Autodesk Fusion 360 part; units mm, degrees
(part 2 of 2)
sketch "Sketch18" plane through (0, 10, 0) normal (0, 1, 0) x (-1, 0, 0)
  line L0 (-0.4884, 10.35) -> (2.2056, 10.35)
  line L1 (2.2056, 10.35) -> (2.2056, 6.15)
  line L2 (2.2056, 6.15) -> (-0.4884, 6.15)
  line L3 (-0.4884, 6.15) -> (-0.4884, 10.35)
  line L4 (-47.1, 4.15) -> (-47.1, 3)
  arc A0 (-47.1, 3) -> (-44.1, 0) centre (-44.1, 3) ccw
  line L5 (-44.1, 0) -> (-5.0797, 0)
  arc A1 (-5.0797, 0) -> (-2.1135, 2.5506) centre (-5.0797, 3) ccw
  line L6 (-2.1135, 2.5506) -> (-1.8712, 4.15)
  line L7 (-1.8712, 4.15) -> (1.2056, 4.15)
  line L8 (1.2056, 4.15) -> (1.2056, -1.7)
  line L9 (1.2056, -1.7) -> (0.2056, -1.7)
  line L10 (0.2056, -1.7) -> (2.7056, -6)
  line L11 (2.7056, -6) -> (2.7056, 4.15)
  line L12 (2.7056, 4.15) -> (3.2056, 4.15)
  line L13 (3.2056, 4.15) -> (3.2056, 12.35)
  line L14 (3.2056, 12.35) -> (-0.6288, 12.35)
  line L15 (-0.6288, 12.35) -> (-0.5226, 13.0506)
  arc A2 (-0.5226, 13.0506) -> (-3.4888, 16.5) centre (-3.4888, 13.5) ccw
  line L16 (-3.4888, 16.5) -> (-44.1, 16.5)
  arc A3 (-44.1, 16.5) -> (-47.1, 13.5) centre (-44.1, 13.5) ccw
  line L17 (-47.1, 13.5) -> (-47.1, 12.35)
  line L18 (-47.1, 12.35) -> (-50.7944, 12.35)
  line L19 (-50.7944, 12.35) -> (-50.7944, 4.15)
  line L20 (-50.7944, 4.15) -> (-50.2944, 4.15)
  line L21 (-50.2944, 4.15) -> (-50.2944, -6)
  line L22 (-50.2944, -6) -> (-47.7944, -1.7)
  line L23 (-47.7944, -1.7) -> (-48.7944, -1.7)
  line L24 (-48.7944, -1.7) -> (-48.7944, 4.15)
  line L25 (-48.7944, 4.15) -> (-47.1, 4.15)
  line L26 (-47.1, 6.15) -> (-49.7944, 6.15)
  line L27 (-49.7944, 6.15) -> (-49.7944, 10.35)
  line L28 (-49.7944, 10.35) -> (-47.1, 10.35)
  line L29 (-47.1, 10.35) -> (-47.1, 6.15)
  line L30 (-26.405, 10.29) -> (-26.405, 11.29)
  line L31 (-26.405, 11.29) -> (-24.005, 11.29)
  line L32 (-24.005, 11.29) -> (-24.005, 10.29)
  line L33 (-24.005, 10.29) -> (-26.405, 10.29)
  line L34 (-22.595, 10.29) -> (-22.595, 11.29)
  line L35 (-22.595, 11.29) -> (-20.195, 11.29)
  line L36 (-20.195, 11.29) -> (-20.195, 10.29)
  line L37 (-20.195, 10.29) -> (-22.595, 10.29)
  line L38 (-11.165, 10.29) -> (-11.165, 11.29)
  line L39 (-11.165, 11.29) -> (-8.765, 11.29)
  line L40 (-8.765, 11.29) -> (-8.765, 10.29)
  line L41 (-8.765, 10.29) -> (-11.165, 10.29)
  line L42 (-39.245, 11.29) -> (-39.245, 10.29)
  line L43 (-39.245, 10.29) -> (-41.645, 10.29)
  line L44 (-41.645, 10.29) -> (-41.645, 11.29)
  line L45 (-41.645, 11.29) -> (-39.245, 11.29)
  line L46 (-37.34, 6.21) -> (-37.34, 5.21)
  line L47 (-37.34, 5.21) -> (-39.74, 5.21)
  line L48 (-39.74, 5.21) -> (-39.74, 6.21)
  line L49 (-39.74, 6.21) -> (-37.34, 6.21)
  line L50 (-3.05, 6.21) -> (-3.05, 5.21)
  line L51 (-3.05, 5.21) -> (-5.45, 5.21)
  line L52 (-5.45, 5.21) -> (-5.45, 6.21)
  line L53 (-5.45, 6.21) -> (-3.05, 6.21)
  line L54 (-6.86, 6.21) -> (-6.86, 5.21)
  line L55 (-6.86, 5.21) -> (-9.26, 5.21)
  line L56 (-9.26, 5.21) -> (-9.26, 6.21)
  line L57 (-9.26, 6.21) -> (-6.86, 6.21)
  line L58 (-10.67, 6.21) -> (-10.67, 5.21)
  line L59 (-10.67, 5.21) -> (-13.07, 5.21)
  line L60 (-13.07, 5.21) -> (-13.07, 6.21)
  line L61 (-13.07, 6.21) -> (-10.67, 6.21)
  line L62 (-30.215, 10.29) -> (-30.215, 11.29)
  line L63 (-30.215, 11.29) -> (-27.815, 11.29)
  line L64 (-27.815, 11.29) -> (-27.815, 10.29)
  line L65 (-27.815, 10.29) -> (-30.215, 10.29)
  line L66 (-18.785, 10.29) -> (-18.785, 11.29)
  line L67 (-18.785, 11.29) -> (-16.385, 11.29)
  line L68 (-16.385, 11.29) -> (-16.385, 10.29)
  line L69 (-16.385, 10.29) -> (-18.785, 10.29)
  line L70 (-14.975, 10.29) -> (-14.975, 11.29)
  line L71 (-14.975, 11.29) -> (-12.575, 11.29)
  line L72 (-12.575, 11.29) -> (-12.575, 10.29)
  line L73 (-12.575, 10.29) -> (-14.975, 10.29)
  line L74 (-34.025, 10.29) -> (-34.025, 11.29)
  line L75 (-34.025, 11.29) -> (-31.625, 11.29)
  line L76 (-31.625, 11.29) -> (-31.625, 10.29)
  line L77 (-31.625, 10.29) -> (-34.025, 10.29)
  line L78 (-25.91, 6.21) -> (-25.91, 5.21)
  line L79 (-25.91, 5.21) -> (-28.31, 5.21)
  line L80 (-28.31, 5.21) -> (-28.31, 6.21)
  line L81 (-28.31, 6.21) -> (-25.91, 6.21)
  line L82 (-18.29, 6.21) -> (-18.29, 5.21)
  line L83 (-18.29, 5.21) -> (-20.69, 5.21)
  line L84 (-20.69, 5.21) -> (-20.69, 6.21)
  line L85 (-20.69, 6.21) -> (-18.29, 6.21)
  line L86 (-33.53, 6.21) -> (-33.53, 5.21)
  line L87 (-33.53, 5.21) -> (-35.93, 5.21)
  line L88 (-35.93, 5.21) -> (-35.93, 6.21)
  line L89 (-35.93, 6.21) -> (-33.53, 6.21)
  line L90 (-41.15, 6.21) -> (-41.15, 5.21)
  line L91 (-41.15, 5.21) -> (-43.55, 5.21)
  line L92 (-43.55, 5.21) -> (-43.55, 6.21)
  line L93 (-43.55, 6.21) -> (-41.15, 6.21)
  line L94 (-14.48, 6.21) -> (-14.48, 5.21)
  line L95 (-14.48, 5.21) -> (-16.88, 5.21)
  line L96 (-16.88, 5.21) -> (-16.88, 6.21)
  line L97 (-16.88, 6.21) -> (-14.48, 6.21)
  line L98 (-37.835, 10.29) -> (-37.835, 11.29)
  line L99 (-37.835, 11.29) -> (-35.435, 11.29)
  line L100 (-35.435, 11.29) -> (-35.435, 10.29)
  line L101 (-35.435, 10.29) -> (-37.835, 10.29)
  line L102 (-7.355, 10.29) -> (-7.355, 11.29)
  line L103 (-7.355, 11.29) -> (-4.955, 11.29)
  line L104 (-4.955, 11.29) -> (-4.955, 10.29)
  line L105 (-4.955, 10.29) -> (-7.355, 10.29)
  line L106 (-29.72, 6.21) -> (-29.72, 5.21)
  line L107 (-29.72, 5.21) -> (-32.12, 5.21)
  line L108 (-32.12, 5.21) -> (-32.12, 6.21)
  line L109 (-32.12, 6.21) -> (-29.72, 6.21)
  line L110 (-22.1, 6.21) -> (-22.1, 5.21)
  line L111 (-22.1, 5.21) -> (-24.5, 5.21)
  line L112 (-24.5, 5.21) -> (-24.5, 6.21)
  line L113 (-24.5, 6.21) -> (-22.1, 6.21)
  line L114 (-42.35, 5.21) -> (-42.35, 0) construction
  line L115 (-43.05, 5.21) -> (-43.05, 0)
  line L116 (-41.65, 5.21) -> (-41.65, 0)
  line L117 (-37.84, 5.21) -> (-37.84, 0)
  line L118 (-39.24, 5.21) -> (-39.24, 0)
  line L119 (-34.03, 5.21) -> (-34.03, 0)
  line L120 (-35.43, 5.21) -> (-35.43, 0)
  line L121 (-30.22, 5.21) -> (-30.22, 0)
  line L122 (-31.62, 5.21) -> (-31.62, 0)
  line L123 (-26.41, 5.21) -> (-26.41, 0)
  line L124 (-27.81, 5.21) -> (-27.81, 0)
  line L125 (-22.6, 5.21) -> (-22.6, 0)
  line L126 (-24, 5.21) -> (-24, 0)
  line L127 (-18.79, 5.21) -> (-18.79, 0)
  line L128 (-20.19, 5.21) -> (-20.19, 0)
  line L129 (-14.98, 5.21) -> (-14.98, 0)
  line L130 (-16.38, 5.21) -> (-16.38, 0)
  line L131 (-11.17, 5.21) -> (-11.17, 0)
  line L132 (-12.57, 5.21) -> (-12.57, 0)
  line L133 (-7.36, 5.21) -> (-7.36, 0)
  line L134 (-8.76, 5.21) -> (-8.76, 0)
  line L135 (-3.55, 5.21) -> (-3.55, 0)
  line L136 (-4.95, 5.21) -> (-4.95, 0)
  line L137 (-3.55, 0) -> (-5.0797, 0)
  dimension "d118" = 0.7
  dimension "d119" = -0.7
  dimension "d122" = 3.81
  dimension "d123" = 0
  constraint midpoint L91 L114.start
  constraint coincident L5 L114.end
  constraint perpendicular L5 L114
  constraint coincident L5.end A1.start
  constraint tangent A1 L137
extrude "Extrude14" add sketch "Sketch18" along normal blind 5.1 contours L5 L91 L115 L116 | L5 L47 L117 L118 | L5 L87 L119 L120 | L5 L107 L121 L122 | L5 L79 L123 L124 | L5 L111 L125 L126 | L5 L83 L127 L128 | L5 L95 L129 L130 | L5 L59 L131 L132 | L5 L55 L133 L134 | A1 L135 L136 L137 | A1 L51 L135 L136 bodies 1
sketch "Sketch20" plane through (43.05, 0, 0) normal (1, 0, 0) x (0, 1, 0)
  line L0 (10, 5.21) -> (10, 0)
  line L1 (10, 0) -> (15.1, 0)
  line L2 (15.1, 0) -> (15.1, 5.21)
  line L3 (15.1, 5.21) -> (10, 5.21)
  line L4 (10, 5.21) -> (14.4, 5.21)
  line L5 (15.1, 4.51) -> (15.1, 2.3)
  arc A0 (15.1, 4.51) -> (14.4, 5.21) centre (14.4, 4.51) ccw
  dimension "d132" = 0.7
  constraint coincident L0.start L3.end
  constraint coincident L2 L5.end
  constraint perpendicular L3 L5
  constraint tangent L4 A0
  constraint tangent L5 A0
  measures "d132" radius of A0
fillet "Fillet9" radius 0.2 11 edges at (42.35, 15.1, 5.21) (38.54, 15.1, 5.21) (34.73, 15.1, 5.21) (30.92, 15.1, 5.21) (27.11, 15.1, 5.21) (23.3, 15.1, 5.21) (19.49, 15.1, 5.21) (15.68, 15.1, 5.21) (11.87, 15.1, 5.21) (8.06, 15.1, 5.21) (4.25, 15.1, 5.21) on bodies 1
sketch "Sketch15" plane through (0, 10, 0) normal (0, 1, 0) x (-1, 0, 0)
  line L0 (-0.4884, 10.35) -> (2.2056, 10.35)
  line L1 (2.2056, 10.35) -> (2.2056, 6.15)
  line L2 (2.2056, 6.15) -> (-0.4884, 6.15)
  line L3 (-0.4884, 6.15) -> (-0.4884, 10.35)
  line L4 (-47.1, 4.15) -> (-47.1, 3)
  arc A0 (-47.1, 3) -> (-44.1, 0) centre (-44.1, 3) ccw
  line L5 (-41.65, 0) -> (-39.24, 0)
  arc A1 (-5.0797, 0) -> (-4.95, 0.0028) centre (-5.0797, 3) ccw
  line L6 (-2.1135, 2.5506) -> (-1.8712, 4.15)
  line L7 (-1.8712, 4.15) -> (1.2056, 4.15)
  line L8 (1.2056, 4.15) -> (1.2056, -1.7)
  line L9 (1.2056, -1.7) -> (0.2056, -1.7)
  line L10 (0.2056, -1.7) -> (2.7056, -6)
  line L11 (2.7056, -6) -> (2.7056, 4.15)
  line L12 (2.7056, 4.15) -> (3.2056, 4.15)
  line L13 (3.2056, 4.15) -> (3.2056, 12.35)
  line L14 (3.2056, 12.35) -> (-0.6288, 12.35)
  line L15 (-0.6288, 12.35) -> (-0.5226, 13.0506)
  arc A2 (-0.5226, 13.0506) -> (-3.4888, 16.5) centre (-3.4888, 13.5) ccw
  line L16 (-3.4888, 16.5) -> (-44.1, 16.5)
  arc A3 (-44.1, 16.5) -> (-47.1, 13.5) centre (-44.1, 13.5) ccw
  line L17 (-47.1, 13.5) -> (-47.1, 12.35)
  line L18 (-47.1, 12.35) -> (-50.7944, 12.35)
  line L19 (-50.7944, 12.35) -> (-50.7944, 4.15)
  line L20 (-50.7944, 4.15) -> (-50.2944, 4.15)
  line L21 (-50.2944, 4.15) -> (-50.2944, -6)
  line L22 (-50.2944, -6) -> (-47.7944, -1.7)
  line L23 (-47.7944, -1.7) -> (-48.7944, -1.7)
  line L24 (-48.7944, -1.7) -> (-48.7944, 4.15)
  line L25 (-48.7944, 4.15) -> (-47.1, 4.15)
  line L26 (-47.1, 6.15) -> (-49.7944, 6.15)
  line L27 (-49.7944, 6.15) -> (-49.7944, 10.35)
  line L28 (-49.7944, 10.35) -> (-47.1, 10.35)
  line L29 (-47.1, 10.35) -> (-47.1, 6.15)
  line L30 (-26.405, 10.29) -> (-26.405, 11.29)
  line L31 (-26.405, 11.29) -> (-24.005, 11.29)
  line L32 (-24.005, 11.29) -> (-24.005, 10.29)
  line L33 (-24.005, 10.29) -> (-26.405, 10.29)
  line L34 (-22.595, 10.29) -> (-22.595, 11.29)
  line L35 (-22.595, 11.29) -> (-20.195, 11.29)
  line L36 (-20.195, 11.29) -> (-20.195, 10.29)
  line L37 (-20.195, 10.29) -> (-22.595, 10.29)
  line L38 (-11.165, 10.29) -> (-11.165, 11.29)
  line L39 (-11.165, 11.29) -> (-8.765, 11.29)
  line L40 (-8.765, 11.29) -> (-8.765, 10.29)
  line L41 (-8.765, 10.29) -> (-11.165, 10.29)
  line L42 (-39.245, 11.29) -> (-39.245, 10.29)
  line L43 (-39.245, 10.29) -> (-41.645, 10.29)
  line L44 (-41.645, 10.29) -> (-41.645, 11.29)
  line L45 (-41.645, 11.29) -> (-39.245, 11.29)
  line L46 (-37.34, 6.21) -> (-37.34, 5.21)
  line L47 (-39.24, 5.21) -> (-39.74, 5.21)
  line L48 (-39.74, 5.21) -> (-39.74, 6.21)
  line L49 (-39.74, 6.21) -> (-37.34, 6.21)
  line L50 (-3.05, 6.21) -> (-3.05, 5.21)
  line L51 (-4.95, 5.21) -> (-5.45, 5.21)
  line L52 (-5.45, 5.21) -> (-5.45, 6.21)
  line L53 (-5.45, 6.21) -> (-3.05, 6.21)
  line L54 (-6.86, 6.21) -> (-6.86, 5.21)
  line L55 (-8.76, 5.21) -> (-9.26, 5.21)
  line L56 (-9.26, 5.21) -> (-9.26, 6.21)
  line L57 (-9.26, 6.21) -> (-6.86, 6.21)
  line L58 (-10.67, 6.21) -> (-10.67, 5.21)
  line L59 (-12.57, 5.21) -> (-13.07, 5.21)
  line L60 (-13.07, 5.21) -> (-13.07, 6.21)
  line L61 (-13.07, 6.21) -> (-10.67, 6.21)
  line L62 (-30.215, 10.29) -> (-30.215, 11.29)
  line L63 (-30.215, 11.29) -> (-27.815, 11.29)
  line L64 (-27.815, 11.29) -> (-27.815, 10.29)
  line L65 (-27.815, 10.29) -> (-30.215, 10.29)
  line L66 (-18.785, 10.29) -> (-18.785, 11.29)
  line L67 (-18.785, 11.29) -> (-16.385, 11.29)
  line L68 (-16.385, 11.29) -> (-16.385, 10.29)
  line L69 (-16.385, 10.29) -> (-18.785, 10.29)
  line L70 (-14.975, 10.29) -> (-14.975, 11.29)
  line L71 (-14.975, 11.29) -> (-12.575, 11.29)
  line L72 (-12.575, 11.29) -> (-12.575, 10.29)
  line L73 (-12.575, 10.29) -> (-14.975, 10.29)
  line L74 (-34.025, 10.29) -> (-34.025, 11.29)
  line L75 (-34.025, 11.29) -> (-31.625, 11.29)
  line L76 (-31.625, 11.29) -> (-31.625, 10.29)
  line L77 (-31.625, 10.29) -> (-34.025, 10.29)
  line L78 (-25.91, 6.21) -> (-25.91, 5.21)
  line L79 (-27.81, 5.21) -> (-28.31, 5.21)
  line L80 (-28.31, 5.21) -> (-28.31, 6.21)
  line L81 (-28.31, 6.21) -> (-25.91, 6.21)
  line L82 (-18.29, 6.21) -> (-18.29, 5.21)
  line L83 (-20.19, 5.21) -> (-20.69, 5.21)
  line L84 (-20.69, 5.21) -> (-20.69, 6.21)
  line L85 (-20.69, 6.21) -> (-18.29, 6.21)
  line L86 (-33.53, 6.21) -> (-33.53, 5.21)
  line L87 (-35.43, 5.21) -> (-35.93, 5.21)
  line L88 (-35.93, 5.21) -> (-35.93, 6.21)
  line L89 (-35.93, 6.21) -> (-33.53, 6.21)
  line L90 (-41.15, 6.21) -> (-41.15, 5.21)
  line L91 (-43.05, 5.21) -> (-43.55, 5.21)
  line L92 (-43.55, 5.21) -> (-43.55, 6.21)
  line L93 (-43.55, 6.21) -> (-41.15, 6.21)
  line L94 (-14.48, 6.21) -> (-14.48, 5.21)
  line L95 (-16.38, 5.21) -> (-16.88, 5.21)
  line L96 (-16.88, 5.21) -> (-16.88, 6.21)
  line L97 (-16.88, 6.21) -> (-14.48, 6.21)
  line L98 (-37.835, 10.29) -> (-37.835, 11.29)
  line L99 (-37.835, 11.29) -> (-35.435, 11.29)
  line L100 (-35.435, 11.29) -> (-35.435, 10.29)
  line L101 (-35.435, 10.29) -> (-37.835, 10.29)
  line L102 (-7.355, 10.29) -> (-7.355, 11.29)
  line L103 (-7.355, 11.29) -> (-4.955, 11.29)
  line L104 (-4.955, 11.29) -> (-4.955, 10.29)
  line L105 (-4.955, 10.29) -> (-7.355, 10.29)
  line L106 (-29.72, 6.21) -> (-29.72, 5.21)
  line L107 (-31.62, 5.21) -> (-32.12, 5.21)
  line L108 (-32.12, 5.21) -> (-32.12, 6.21)
  line L109 (-32.12, 6.21) -> (-29.72, 6.21)
  line L110 (-22.1, 6.21) -> (-22.1, 5.21)
  line L111 (-24, 5.21) -> (-24.5, 5.21)
  line L112 (-24.5, 5.21) -> (-24.5, 6.21)
  line L113 (-24.5, 6.21) -> (-22.1, 6.21)
  line L114 (-41.545, 10.99) -> (-39.345, 10.99)
  line L115 (-39.345, 10.99) -> (-39.345, 10.59)
  line L116 (-39.345, 10.59) -> (-41.545, 10.59)
  line L117 (-41.545, 10.59) -> (-41.545, 10.99)
  line L118 (-41.65, 5.21) -> (-41.65, 0)
  line L119 (-39.24, 0) -> (-39.24, 5.21)
  line L120 (-37.34, 5.21) -> (-37.84, 5.21)
  line L121 (-37.84, 5.21) -> (-37.84, 0)
  line L122 (-37.84, 0) -> (-35.43, 0)
  line L123 (-35.43, 0) -> (-35.43, 5.21)
  line L124 (-33.53, 5.21) -> (-34.03, 5.21)
  line L125 (-34.03, 5.21) -> (-34.03, 0)
  line L126 (-34.03, 0) -> (-31.62, 0)
  line L127 (-31.62, 0) -> (-31.62, 5.21)
  line L128 (-29.72, 5.21) -> (-30.22, 5.21)
  line L129 (-30.22, 5.21) -> (-30.22, 0)
  line L130 (-30.22, 0) -> (-27.81, 0)
  line L131 (-27.81, 0) -> (-27.81, 5.21)
  line L132 (-25.91, 5.21) -> (-26.41, 5.21)
  line L133 (-26.41, 5.21) -> (-26.41, 0)
  line L134 (-26.41, 0) -> (-24, 0)
  line L135 (-24, 0) -> (-24, 5.21)
  line L136 (-22.1, 5.21) -> (-22.6, 5.21)
  line L137 (-22.6, 5.21) -> (-22.6, 0)
  line L138 (-22.6, 0) -> (-20.19, 0)
  line L139 (-20.19, 0) -> (-20.19, 5.21)
  line L140 (-18.29, 5.21) -> (-18.79, 5.21)
  line L141 (-18.79, 5.21) -> (-18.79, 0)
  line L142 (-18.79, 0) -> (-16.38, 0)
  line L143 (-16.38, 0) -> (-16.38, 5.21)
  line L144 (-14.48, 5.21) -> (-14.98, 5.21)
  line L145 (-14.98, 5.21) -> (-14.98, 0)
  line L146 (-14.98, 0) -> (-12.57, 0)
  line L147 (-12.57, 0) -> (-12.57, 5.21)
  line L148 (-10.67, 5.21) -> (-11.17, 5.21)
  line L149 (-11.17, 5.21) -> (-11.17, 0)
  line L150 (-11.17, 0) -> (-8.76, 0)
  line L151 (-8.76, 0) -> (-8.76, 5.21)
  line L152 (-6.86, 5.21) -> (-7.36, 5.21)
  line L153 (-7.36, 5.21) -> (-7.36, 0)
  line L154 (-7.36, 0) -> (-5.0797, 0)
  line L155 (-4.95, 0.0028) -> (-4.95, 5.21)
  line L156 (-3.05, 5.21) -> (-3.55, 5.21)
  line L157 (-3.55, 5.21) -> (-3.55, 0.4193)
  arc A4 (-3.55, 0.4193) -> (-2.1135, 2.5506) centre (-5.0797, 3) ccw
  line L158 (-44.1, 0) -> (-43.05, 0)
  line L159 (-43.05, 0) -> (-43.05, 5.21)
  line L160 (-41.15, 5.21) -> (-41.65, 5.21)
  dimension "d88" = 0.1
  dimension "d89" = 0.1
  dimension "d90" = 0.3
  dimension "d91" = 0.3
  constraint horizontal L114
  constraint vertical L115
  constraint horizontal L116
  constraint vertical L117
  measures "d88" distance of L42 L115
  measures "d89" distance of L44 L117
  measures "d90" distance of L45 L114
  measures "d91" distance of L43 L116
extrude "Extrude11" add sketch "Sketch15" against normal blind 10 separate body contours L114 L115 L116 L117 makes body 2
sketch "Sketch16" plane through (0, 0, 10.99) normal (0, 0, 1) x (-1, 0, 0)
  line L0 (-41.545, -10) -> (-39.345, -10)
  line L1 (-39.345, -10) -> (-39.345, 0)
  line L2 (-39.345, 0) -> (-41.545, 0)
  line L3 (-41.545, 0) -> (-41.545, -10)
  line L4 (-39.745, 0) -> (-41.145, 0)
  line L5 (-41.145, 0) -> (-41.145, -7)
  line L6 (-41.145, -7) -> (-39.745, -7)
  line L7 (-39.745, -7) -> (-39.745, 0)
  dimension "d94" = 7
  dimension "d95" = 0.4
  dimension "d96" = 0.4
  constraint horizontal L4
  constraint vertical L5
  constraint horizontal L6
  constraint vertical L7
  constraint coincident L2 L4.start
  measures "d94" distance of L4.start L6.end
  measures "d95" distance of L1 L7
  measures "d96" distance of L3 L5
extrude "Extrude12" cut sketch "Sketch16" against normal through all contours L2 L4 L5 L6 L7 bodies 2
sketch "Sketch17" plane through (0, 10, 0) normal (0, 1, 0) x (-1, 0, 0)
  line L0 (-41.545, 10.59) -> (-39.345, 10.59)
  line L1 (-39.345, 10.59) -> (-39.345, 10.99)
  line L2 (-39.345, 10.99) -> (-41.545, 10.99)
  line L3 (-41.545, 10.99) -> (-41.545, 10.59)
  line L4 (-41.545, 10.99) -> (-39.345, 10.99)
  line L5 (-39.345, 10.99) -> (-39.345, -4.5)
  line L6 (-39.345, -4.5) -> (-41.545, -4.5)
  line L7 (-41.545, -4.5) -> (-41.545, 10.99)
  line L8 (-40.445, -4.5) -> (-40.445, 10.99) construction
  line L9 (-40.045, -4.5) -> (-40.045, 10.99)
  line L10 (-40.845, -4.5) -> (-40.845, 10.99)
  line L11 (-40.845, 6.71) -> (-41.545, 7.41)
  line L12 (-40.845, 6.71) -> (-39.8551, 6.71) construction
  line L13 (-40.045, 6.71) -> (-39.345, 7.41)
  line L14 (-40.845, 4.71) -> (-41.545, 4.01)
  line L15 (-40.845, 4.71) -> (-39.8551, 4.71) construction
  line L16 (-40.045, 4.71) -> (-39.345, 4.01)
  line L17 (-40.845, 0) -> (-41.545, 0.7)
  line L18 (-40.045, 0) -> (-39.345, 0.7)
  line L19 (-39.645, 10.99) -> (-39.645, -4.5)
  line L20 (-41.245, -4.5) -> (-41.245, 10.99)
  line L21 (-40.445, -4.5) -> (-40.045, -4.1)
  line L22 (-40.445, -4.5) -> (-39.8793, -4.5) construction
  line L23 (-40.445, -4.5) -> (-40.845, -4.1)
  line L24 (-7.36, 0) -> (-5.0797, 0)
  line L25 (-11.17, 0) -> (-8.76, 0)
  line L26 (-14.98, 0) -> (-12.57, 0)
  line L27 (-18.79, 0) -> (-16.38, 0)
  line L28 (-22.6, 0) -> (-20.19, 0)
  line L29 (-26.41, 0) -> (-24, 0)
  line L30 (-30.22, 0) -> (-27.81, 0)
  line L31 (-34.03, 0) -> (-31.62, 0)
  line L32 (-37.84, 0) -> (-35.43, 0)
  line L33 (-41.65, 0) -> (-39.24, 0)
  line L34 (-43.05, 5.21) -> (-43.55, 5.21)
  line L35 (-44.1, 0) -> (-43.05, 0)
  line L36 (-41.15, 5.21) -> (-41.65, 5.21)
  line L37 (-40.845, 10.99) -> (-40.2793, 10.99) construction
  line L38 (-40.845, 10.59) -> (-41.245, 10.19)
  line L39 (-40.845, 10.59) -> (-40.2793, 10.59) construction
  line L40 (-40.045, 10.59) -> (-39.645, 10.19)
  point P0 (-41.15, 6.21)
  dimension "d99" = 0.4
  dimension "d100" = -0.4
  dimension "d101" = 135
  dimension "d102" = 0.5
  dimension "d103" = 135
  dimension "d104" = 0.9899
  dimension "d106" = 0.3
  dimension "d107" = 0.3
  dimension "d110" = 45
  dimension "d158" = 135
  constraint horizontal L4
  constraint vertical L5
  constraint horizontal L6
  constraint vertical L7
  constraint coincident L2.end L3.start
  constraint midpoint L6 L8.start
  constraint midpoint L4 L8.end
  constraint horizontal L12
  constraint coincident L10 L11.start
  constraint coincident L7 L11.end
  constraint coincident L12 L13.start
  constraint coincident L9 L13.start
  constraint coincident L5 L13.end
  constraint perpendicular L11 L13
  constraint horizontal L15
  constraint coincident L10 L14.start
  constraint coincident L7 L14.end
  constraint coincident L9 L16.start
  constraint coincident L15 L16.start
  constraint coincident L5 L16.end
  constraint coincident L10 L17.start
  constraint coincident L7 L17.end
  constraint parallel L16 L17
  constraint coincident L9 L18.start
  constraint coincident L5 L18.end
  constraint perpendicular L17 L18
  constraint horizontal L22
  constraint coincident L9 L21.end
  constraint coincident L10 L23.end
  constraint perpendicular L21 L23
  constraint horizontal L37
  constraint horizontal L39
  constraint coincident L0 L38.start
  constraint coincident L10 L38.start
  constraint coincident L20 L38.end
  constraint coincident L9 L40.start
  constraint coincident L0 L40.start
  constraint coincident L19 L40.end
  constraint perpendicular L38 L40
  measures "d101" angle of L11 L12
  measures "d102" vertical distance of L11.start P0
  measures "d103" angle of L14 L15
  measures "d104" distance of L14.start L15.end
  measures "d110" angle of L21 L22
  measures "d158" angle of L38 L39
extrude "Extrude13" add sketch "Sketch17" along normal blind 0.4 contours L0 L2 L4 L9 L10 | L0 L9 L10 L33 | L10 L11 L20 L38 | L9 L13 L19 L40 | L10 L14 L17 L20 | L9 L16 L18 L19 | L9 L10 L21 L23 L33 bodies 2
fillet "Fillet8" radius 0.2 23 edges at (39.745, 0, 10.79) (41.145, 0, 10.79) (39.345, 10, 10.79) (41.545, 10, 10.79) (40.445, 10.4, 10.99) (39.645, 10.2, 7.11) (40.045, 10.2, 6.71) (40.045, 10.2, 4.71) (39.645, 10.2, 4.31) (41.245, 10.2, 7.11) (40.845, 10.2, 6.71) (40.845, 10.2, 4.71) (41.245, 10.2, 4.31) (41.245, 10.2, 0.4) (39.645, 10.2, 0.4) (40.045, 10.2, -4.1) (40.845, 10.2, -4.1) (41.245, 10.2, 10.19) (40.845, 10.2, 10.59) (39.645, 10.2, 10.19) (40.045, 10.2, 10.59) (40.845, 10.2, 0) (40.045, 10.2, 0) on bodies 2
pattern_linear "R-Pattern1" count 10 spacing 3.81 along (-1, 0, 0) of bodies 2 makes body 3 at (36.3683, 10.4, 2.9791) makes body 4 at (32.5583, 10.4, 2.9791) makes body 5 at (28.7483, 10.4, 2.9791) makes body 6 at (24.9383, 10.4, 2.9791) makes body 7 at (21.1283, 10.4, 2.9791) makes body 8 at (17.3183, 10.4, 2.9791) makes body 9 at (13.5083, 10.4, 2.9791) makes body 10 at (9.6983, 10.4, 2.9791) makes body 11 at (5.8883, 10.4, 2.9791)
sketch "Sketch19" plane through (0, 10, 0) normal (0, 1, 0) x (-1, 0, 0)
  line L0 (-41.65, 5.21) -> (-41.65, 0)
  line L1 (-41.65, 0) -> (-39.24, 0)
  line L2 (-39.24, 0) -> (-39.24, 5.21)
  line L3 (-39.24, 5.21) -> (-39.74, 5.21)
  line L4 (-39.74, 5.21) -> (-39.74, 6.21)
  line L5 (-39.74, 6.21) -> (-37.34, 6.21)
  line L6 (-37.34, 6.21) -> (-37.34, 5.21)
  line L7 (-37.34, 5.21) -> (-37.84, 5.21)
  line L8 (-37.84, 5.21) -> (-37.84, 0)
  line L9 (-37.84, 0) -> (-35.43, 0)
  line L10 (-35.43, 0) -> (-35.43, 5.21)
  line L11 (-35.43, 5.21) -> (-35.93, 5.21)
  line L12 (-35.93, 5.21) -> (-35.93, 6.21)
  line L13 (-35.93, 6.21) -> (-33.53, 6.21)
  line L14 (-33.53, 6.21) -> (-33.53, 5.21)
  line L15 (-33.53, 5.21) -> (-34.03, 5.21)
  line L16 (-34.03, 5.21) -> (-34.03, 0)
  line L17 (-34.03, 0) -> (-31.62, 0)
  line L18 (-31.62, 0) -> (-31.62, 5.21)
  line L19 (-31.62, 5.21) -> (-32.12, 5.21)
  line L20 (-32.12, 5.21) -> (-32.12, 6.21)
  line L21 (-32.12, 6.21) -> (-29.72, 6.21)
  line L22 (-29.72, 6.21) -> (-29.72, 5.21)
  line L23 (-29.72, 5.21) -> (-30.22, 5.21)
  line L24 (-30.22, 5.21) -> (-30.22, 0)
  line L25 (-30.22, 0) -> (-27.81, 0)
  line L26 (-27.81, 0) -> (-27.81, 5.21)
  line L27 (-27.81, 5.21) -> (-28.31, 5.21)
  line L28 (-28.31, 5.21) -> (-28.31, 6.21)
  line L29 (-28.31, 6.21) -> (-25.91, 6.21)
  line L30 (-25.91, 6.21) -> (-25.91, 5.21)
  line L31 (-25.91, 5.21) -> (-26.41, 5.21)
  line L32 (-26.41, 5.21) -> (-26.41, 0)
  line L33 (-26.41, 0) -> (-24, 0)
  line L34 (-24, 0) -> (-24, 5.21)
  line L35 (-24, 5.21) -> (-24.5, 5.21)
  line L36 (-24.5, 5.21) -> (-24.5, 6.21)
  line L37 (-24.5, 6.21) -> (-22.1, 6.21)
  line L38 (-22.1, 6.21) -> (-22.1, 5.21)
  line L39 (-22.1, 5.21) -> (-22.6, 5.21)
  line L40 (-22.6, 5.21) -> (-22.6, 0)
  line L41 (-22.6, 0) -> (-20.19, 0)
  line L42 (-20.19, 0) -> (-20.19, 5.21)
  line L43 (-20.19, 5.21) -> (-20.69, 5.21)
  line L44 (-20.69, 5.21) -> (-20.69, 6.21)
  line L45 (-20.69, 6.21) -> (-18.29, 6.21)
  line L46 (-18.29, 6.21) -> (-18.29, 5.21)
  line L47 (-18.29, 5.21) -> (-18.79, 5.21)
  line L48 (-18.79, 5.21) -> (-18.79, 0)
  line L49 (-18.79, 0) -> (-16.38, 0)
  line L50 (-16.38, 0) -> (-16.38, 5.21)
  line L51 (-16.38, 5.21) -> (-16.88, 5.21)
  line L52 (-16.88, 5.21) -> (-16.88, 6.21)
  line L53 (-16.88, 6.21) -> (-14.48, 6.21)
  line L54 (-14.48, 6.21) -> (-14.48, 5.21)
  line L55 (-14.48, 5.21) -> (-14.98, 5.21)
  line L56 (-14.98, 5.21) -> (-14.98, 0)
  line L57 (-14.98, 0) -> (-12.57, 0)
  line L58 (-12.57, 0) -> (-12.57, 5.21)
  line L59 (-12.57, 5.21) -> (-13.07, 5.21)
  line L60 (-13.07, 5.21) -> (-13.07, 6.21)
  line L61 (-13.07, 6.21) -> (-10.67, 6.21)
  line L62 (-10.67, 6.21) -> (-10.67, 5.21)
  line L63 (-10.67, 5.21) -> (-11.17, 5.21)
  line L64 (-11.17, 5.21) -> (-11.17, 0)
  line L65 (-11.17, 0) -> (-8.76, 0)
  line L66 (-8.76, 0) -> (-8.76, 5.21)
  line L67 (-8.76, 5.21) -> (-9.26, 5.21)
  line L68 (-9.26, 5.21) -> (-9.26, 6.21)
  line L69 (-9.26, 6.21) -> (-6.86, 6.21)
  line L70 (-6.86, 6.21) -> (-6.86, 5.21)
  line L71 (-6.86, 5.21) -> (-7.36, 5.21)
  line L72 (-7.36, 5.21) -> (-7.36, 0)
  line L73 (-7.36, 0) -> (-5.0797, 0)
  arc A0 (-5.0797, 0) -> (-4.95, 0.0028) centre (-5.0797, 3) ccw
  line L74 (-4.95, 0.0028) -> (-4.95, 5.21)
  line L75 (-4.95, 5.21) -> (-5.45, 5.21)
  line L76 (-5.45, 5.21) -> (-5.45, 6.21)
  line L77 (-5.45, 6.21) -> (-3.05, 6.21)
  line L78 (-3.05, 6.21) -> (-3.05, 5.21)
  line L79 (-3.05, 5.21) -> (-3.55, 5.21)
  line L80 (-3.55, 5.21) -> (-3.55, 0.4193)
  arc A1 (-3.55, 0.4193) -> (-2.1135, 2.5506) centre (-5.0797, 3) ccw
  line L81 (-2.1135, 2.5506) -> (-1.8712, 4.15)
  line L82 (-1.8712, 4.15) -> (1.2056, 4.15)
  line L83 (1.2056, 4.15) -> (1.2056, -1.7)
  line L84 (1.2056, -1.7) -> (0.2056, -1.7)
  line L85 (0.2056, -1.7) -> (2.7056, -6)
  line L86 (2.7056, -6) -> (2.7056, 4.15)
  line L87 (2.7056, 4.15) -> (3.2056, 4.15)
  line L88 (3.2056, 4.15) -> (3.2056, 12.35)
  line L89 (3.2056, 12.35) -> (-0.6288, 12.35)
  line L90 (-0.6288, 12.35) -> (-0.5226, 13.0506)
  arc A2 (-0.5226, 13.0506) -> (-3.4888, 16.5) centre (-3.4888, 13.5) ccw
  line L91 (-3.4888, 16.5) -> (-44.1, 16.5)
  arc A3 (-44.1, 16.5) -> (-47.1, 13.5) centre (-44.1, 13.5) ccw
  line L92 (-47.1, 13.5) -> (-47.1, 12.35)
  line L93 (-47.1, 12.35) -> (-50.7944, 12.35)
  line L94 (-50.7944, 12.35) -> (-50.7944, 4.15)
  line L95 (-50.7944, 4.15) -> (-50.2944, 4.15)
  line L96 (-50.2944, 4.15) -> (-50.2944, -6)
  line L97 (-50.2944, -6) -> (-47.7944, -1.7)
  line L98 (-47.7944, -1.7) -> (-48.7944, -1.7)
  line L99 (-48.7944, -1.7) -> (-48.7944, 4.15)
  line L100 (-48.7944, 4.15) -> (-47.1, 4.15)
  line L101 (-47.1, 4.15) -> (-47.1, 3)
  arc A4 (-47.1, 3) -> (-44.1, 0) centre (-44.1, 3) ccw
  line L102 (-44.1, 0) -> (-43.05, 0)
  line L103 (-43.05, 0) -> (-43.05, 5.21)
  line L104 (-43.05, 5.21) -> (-43.55, 5.21)
  line L105 (-43.55, 5.21) -> (-43.55, 6.21)
  line L106 (-43.55, 6.21) -> (-41.15, 6.21)
  line L107 (-41.15, 6.21) -> (-41.15, 5.21)
  line L108 (-41.15, 5.21) -> (-41.65, 5.21)
  line L109 (-0.4884, 10.35) -> (2.2056, 10.35)
  line L110 (2.2056, 10.35) -> (2.2056, 6.15)
  line L111 (2.2056, 6.15) -> (-0.4884, 6.15)
  line L112 (-0.4884, 6.15) -> (-0.4884, 10.35)
  line L113 (-47.1, 6.15) -> (-49.7944, 6.15)
  line L114 (-49.7944, 6.15) -> (-49.7944, 10.35)
  line L115 (-49.7944, 10.35) -> (-47.1, 10.35)
  line L116 (-47.1, 10.35) -> (-47.1, 6.15)
  line L117 (-26.405, 10.29) -> (-26.405, 11.29)
  line L118 (-26.405, 11.29) -> (-24.005, 11.29)
  line L119 (-24.005, 11.29) -> (-24.005, 10.29)
  line L120 (-24.005, 10.29) -> (-26.405, 10.29)
  line L121 (-22.595, 10.29) -> (-22.595, 11.29)
  line L122 (-22.595, 11.29) -> (-20.195, 11.29)
  line L123 (-20.195, 11.29) -> (-20.195, 10.29)
  line L124 (-20.195, 10.29) -> (-22.595, 10.29)
  line L125 (-11.165, 10.29) -> (-11.165, 11.29)
  line L126 (-11.165, 11.29) -> (-8.765, 11.29)
  line L127 (-8.765, 11.29) -> (-8.765, 10.29)
  line L128 (-8.765, 10.29) -> (-11.165, 10.29)
  line L129 (-39.245, 11.29) -> (-39.245, 10.29)
  line L130 (-39.245, 10.29) -> (-41.645, 10.29)
  line L131 (-41.645, 10.29) -> (-41.645, 11.29)
  line L132 (-41.645, 11.29) -> (-39.245, 11.29)
  line L133 (-30.215, 10.29) -> (-30.215, 11.29)
  line L134 (-30.215, 11.29) -> (-27.815, 11.29)
  line L135 (-27.815, 11.29) -> (-27.815, 10.29)
  line L136 (-27.815, 10.29) -> (-30.215, 10.29)
  line L137 (-18.785, 10.29) -> (-18.785, 11.29)
  line L138 (-18.785, 11.29) -> (-16.385, 11.29)
  line L139 (-16.385, 11.29) -> (-16.385, 10.29)
  line L140 (-16.385, 10.29) -> (-18.785, 10.29)
  line L141 (-14.975, 10.29) -> (-14.975, 11.29)
  line L142 (-14.975, 11.29) -> (-12.575, 11.29)
  line L143 (-12.575, 11.29) -> (-12.575, 10.29)
  line L144 (-12.575, 10.29) -> (-14.975, 10.29)
  line L145 (-34.025, 10.29) -> (-34.025, 11.29)
  line L146 (-34.025, 11.29) -> (-31.625, 11.29)
  line L147 (-31.625, 11.29) -> (-31.625, 10.29)
  line L148 (-31.625, 10.29) -> (-34.025, 10.29)
  line L149 (-37.835, 10.29) -> (-37.835, 11.29)
  line L150 (-37.835, 11.29) -> (-35.435, 11.29)
  line L151 (-35.435, 11.29) -> (-35.435, 10.29)
  line L152 (-35.435, 10.29) -> (-37.835, 10.29)
  line L153 (-7.355, 10.29) -> (-7.355, 11.29)
  line L154 (-7.355, 11.29) -> (-4.955, 11.29)
  line L155 (-4.955, 11.29) -> (-4.955, 10.29)
  line L156 (-4.955, 10.29) -> (-7.355, 10.29)
  line L157 (-43.45, 5.91) -> (-41.25, 5.91)
  line L158 (-41.25, 5.91) -> (-41.25, 5.51)
  line L159 (-41.25, 5.51) -> (-43.45, 5.51)
  line L160 (-43.45, 5.51) -> (-43.45, 5.91)
  dimension "d126" = 0.1
  dimension "d127" = 0.1
  dimension "d128" = 0.3
  dimension "d129" = 0.3
  constraint horizontal L157
  constraint vertical L158
  constraint horizontal L159
  constraint vertical L160
  measures "d126" distance of L107 L158
  measures "d127" distance of L105 L160
  measures "d128" distance of L106 L157
  measures "d129" distance of L104 L159
extrude "Extrude15" add sketch "Sketch19" along normal blind 5.1 and the other way blind 10 separate body contours L157 L158 L159 L160 makes body 12
sketch "Sketch23" plane through (0, 0, 5.91) normal (0, 0, 1) x (-1, 0, 0)
  line L0 (-43.45, 0) -> (-43.45, -15.1)
  line L1 (-43.45, -15.1) -> (-41.25, -15.1)
  line L2 (-41.25, -15.1) -> (-41.25, 0)
  line L3 (-41.25, 0) -> (-43.45, 0)
  line L4 (-41.65, 0) -> (-43.05, 0)
  line L5 (-43.05, 0) -> (-43.05, -7)
  line L6 (-43.05, -7) -> (-41.65, -7)
  line L7 (-41.65, -7) -> (-41.65, 0)
  line L8 (-43.45, -8.6) -> (-41.25, -8.6)
  line L9 (-42.35, -8.6) -> (-42.35, -15.1) construction
  line L10 (-42.75, -8.6) -> (-42.75, -15.1)
  line L11 (-41.95, -8.6) -> (-41.95, -15.1)
  line L12 (-43.25, 0) -> (-43.25, -15.1)
  line L13 (-41.45, -15.1) -> (-41.45, 0)
  line L14 (-42.75, -9.4) -> (-43.25, -9.9)
  line L15 (-42.75, -9.4) -> (-41.95, -9.4) construction
  line L16 (-41.95, -9.4) -> (-41.45, -9.9)
  line L17 (-41.95, -14.7) -> (-41.45, -14.2)
  line L18 (-41.95, -14.7) -> (-41.2429, -14.7) construction
  line L19 (-42.75, -14.6825) -> (-43.25, -14.1825)
  dimension "d143" = 7
  dimension "d144" = 0.4
  dimension "d145" = 0.4
  dimension "d147" = 6.5
  dimension "d148" = 0.4
  dimension "d149" = -0.4
  dimension "d150" = -0.2
  dimension "d151" = -0.2
  dimension "d152" = 135
  dimension "d153" = 0.8
  dimension "d154" = 45
  dimension "d155" = 0.4
  constraint horizontal L4
  constraint vertical L5
  constraint horizontal L6
  constraint vertical L7
  constraint coincident L3 L4.start
  constraint midpoint L8 L9.start
  constraint midpoint L1 L9.end
  constraint perpendicular L1 L9
  constraint parallel L1 L8
  constraint horizontal L15
  constraint coincident L10 L14.start
  constraint coincident L12 L14.end
  constraint coincident L11 L15.end
  constraint coincident L13 L16.end
  constraint horizontal L18
  constraint coincident L11 L17.start
  constraint coincident L13 L17.end
  constraint coincident L10 L19.start
  constraint coincident L12 L19.end
  constraint perpendicular L17 L19
  measures "d143" distance of L4.end L5.end
  measures "d144" distance of L0 L5
  measures "d145" distance of L2 L7
  measures "d147" distance of L1 L8
  measures "d152" angle of L14 L15
  measures "d153" distance of L8 L15
  measures "d154" angle of L17 L18
  measures "d155" distance of L11.end L17.start
extrude "Extrude19" cut sketch "Sketch23" against normal through all contours L0 L1 L8 L12 | L8 L10 L12 L14 | L3 L4 L5 L6 L7 | L1 L10 L12 L19 | L8 L11 L13 L16 | L1 L11 L13 L17 | L1 L2 L8 L13 bodies 12
sketch "Sketch24" plane through (0, 15.1, 0) normal (0, 1, 0) x (-1, 0, 0)
  line L0 (-41.95, 5.51) -> (-41.95, 5.91)
  line L1 (-41.95, 5.91) -> (-42.75, 5.91)
  line L2 (-42.75, 5.91) -> (-42.75, 5.51)
  line L3 (-42.75, 5.51) -> (-41.95, 5.51)
  line L4 (-42.75, 5.91) -> (-41.95, 5.91)
  line L5 (-41.95, 5.91) -> (-41.95, -4.5)
  line L6 (-41.95, -4.5) -> (-42.75, -4.5)
  line L7 (-42.75, -4.5) -> (-42.75, 5.91)
  line L8 (-43.05, 0) -> (-41.65, 0)
  line L9 (-42.35, -4.5) -> (-42.35, 5.91) construction
  line L10 (-41.65, 5.91) -> (-41.65, -4.5)
  line L11 (-43.05, -4.5) -> (-43.05, 5.91)
  line L12 (-41.95, 4.81) -> (-41.65, 4.51)
  line L13 (-41.95, 4.81) -> (-41.5257, 4.81) construction
  line L14 (-42.75, 4.81) -> (-43.05, 4.51)
  line L15 (-42.75, 4.81) -> (-41.95, 4.81) construction
  line L16 (-41.95, 0) -> (-41.65, 0.3)
  line L17 (-41.95, 0) -> (-41.5257, 0) construction
  line L18 (-42.75, 0) -> (-43.05, 0.3)
  line L19 (-42.35, -4.5) -> (-41.95, -4.1)
  line L20 (-42.35, -4.5) -> (-41.7843, -4.5) construction
  line L21 (-42.35, -4.5) -> (-42.75, -4.1)
  dimension "d159" = 4.5
  dimension "d160" = -0.3
  dimension "d161" = -0.3
  dimension "d162" = 45
  dimension "d163" = 135
  dimension "d164" = 1.1
  dimension "d165" = 45
  dimension "d166" = 45
  constraint horizontal L4
  constraint vertical L5
  constraint horizontal L6
  constraint vertical L7
  constraint coincident L1.end L2.start
  constraint midpoint L6 L9.start
  constraint midpoint L4 L9.end
  constraint horizontal L13
  constraint coincident L5 L12.start
  constraint coincident L10 L12.end
  constraint horizontal L15
  constraint coincident L7 L14.start
  constraint coincident L11 L14.end
  constraint horizontal L17
  constraint coincident L8 L16.start
  constraint coincident L5 L16.start
  constraint coincident L10 L16.end
  constraint coincident L8 L18.start
  constraint coincident L7 L18.start
  constraint coincident L11 L18.end
  constraint perpendicular L16 L18
  constraint horizontal L20
  constraint coincident L5 L19.end
  constraint coincident L7 L21.end
  constraint perpendicular L19 L21
  measures "d159" distance of L6 L8
  measures "d162" angle of L12 L13
  measures "d163" angle of L14 L15
  measures "d164" distance of L0.end L12.start
  measures "d165" angle of L16 L17
  measures "d166" angle of L19 L20
extrude "Extrude20" add sketch "Sketch24" along normal blind 0.4 contours L0 L1 L2 L3 L4 L5 L7 | L3 L5 L7 L8 | L5 L10 L12 L16 | L7 L11 L14 L18 | L5 L7 L8 L19 L21 bodies 12
fillet "Fillet10" radius 0.2 25 edges at (41.65, 0, 5.71) (43.05, 0, 5.71) (43.45, 8.6, 5.71) (41.25, 8.6, 5.71) (42.75, 8.6, 5.71) (41.95, 8.6, 5.71) (41.95, 9.4, 5.71) (41.45, 9.9, 5.71) (42.75, 9.4, 5.71) (43.25, 9.9, 5.71) (43.25, 14.1825, 5.71) (42.75, 14.6825, 5.71) (42.75, 15.3, 4.81) (43.05, 15.3, 4.51) (41.45, 14.2, 5.71) (41.95, 14.7, 5.71) (41.95, 15.3, 4.81) (41.65, 15.3, 4.51) (41.65, 15.3, 0.3) (41.95, 15.3, 0) (42.75, 15.3, 0) (43.05, 15.3, 0.3) (42.75, 15.3, -4.1) (41.95, 15.3, -4.1) (42.35, 15.5, 5.91) on bodies 12
pattern_linear "R-Pattern2" count 11 spacing 3.81 along (-1, 0, 0) of bodies 12 makes body 13 at (38.24, 12.7332, 5.91) makes body 14 at (34.43, 12.7332, 5.91) makes body 15 at (30.62, 12.7332, 5.91) makes body 16 at (26.81, 12.7332, 5.91) makes body 17 at (23, 12.7332, 5.91) makes body 18 at (19.19, 12.7332, 5.91) makes body 19 at (15.38, 12.7332, 5.91) makes body 20 at (11.57, 12.7332, 5.91) makes body 21 at (7.76, 12.7332, 5.91) makes body 22 at (3.95, 12.7332, 5.91)
fillet "Fillet5" radius 0.2 113 edges at (1.2141, 0, 15.456) (23.7944, 0, 16.5) (46.2213, 0, 15.6213) (47.1, 0, 8.25) (46.2213, 0, 0.8787) (24.5898, 0, 0) (3.1237, 0, 0.7253) (1.3181, 0, 7.8006) (1.8897, 0, 14.7409) (23.7944, 0, 15.5241) (45.5312, 0, 14.9312) (46.1241, 0, 8.25) (45.5312, 0, 1.5688) (24.525, 0, 0.9759) (3.8893, 0, 1.4153) (3.45, 0, 3.843) (47.1, 10, 12.925) (46.2213, 10, 15.6213) (23.7944, 10, 16.5) (1.2141, 10, 15.456) (0.5757, 10, 12.7003) (48.9472, 10, 12.35) (48.9472, 6.7, 12.35) (48.4472, 6.7, 10.35) (47.1, 8.35, 12.35) (47.1, 6.7, 11.35) (50.7944, 8.35, 12.35) (50.7944, 10, 8.25) (50.7944, 6.7, 8.25) (49.7944, 6.7, 8.25) (48.4472, 6.7, 6.15) (47.1, 8.35, 6.15) (47.1, 6.7, 5.15) (47.9472, 6.7, 4.15) (50.7944, 8.35, 4.15) (50.2944, 6.7, -0.925) (48.7944, 6.7, 1.225) (48.2944, 6.7, -1.7) (49.0444, 6.7, -3.85) (50.2944, 10, -0.925) (50.2944, 8.35, -6) (47.7944, 8.35, -1.7) (48.7944, 10, 1.225) (48.2944, 10, -1.7) (49.0444, 10, -3.85) (47.9472, 10, 4.15) (48.4472, 10, 6.15) (49.7944, 10, 8.25) (48.4472, 10, 10.35) (49.7944, 8.35, 10.35) (47.1, 10, 8.25) (49.7944, 8.35, 6.15) (1.9924, 10, 3.3503) (2.592, 10, 1.3233) (5.0148, 10, 0.0007) (43.575, 10, 0) (6.2198, 10, 0) (9.965, 10, 0) (13.775, 10, 0) (17.585, 10, 0) (21.395, 10, 0) (25.205, 10, 0) (29.015, 10, 0) (32.825, 10, 0) (36.635, 10, 0) (40.445, 10, 0) (46.2213, 10, 0.8787) (47.1, 10, 3.575) (-1.2884, 10, 12.35) (-1.2884, 6.7, 12.35) (0.6288, 8.35, 12.35) (-3.2056, 8.35, 12.35) (-3.2056, 10, 8.25) (-3.2056, 6.7, 8.25) (-0.8586, 10, 10.35) (-2.2056, 10, 8.25) (-0.8586, 10, 6.15) (0.4884, 10, 8.25) (0.4884, 6.7, 8.25) (-0.8586, 6.7, 6.15) (0.3328, 10, 4.15) (-1.2056, 10, 1.225) (-2.7056, 10, -0.925) (-2.7056, 6.7, -0.925) (-0.2056, 8.35, -1.7) (-0.7056, 10, -1.7) (-1.4556, 10, -3.85) (-2.7056, 8.35, -6) (0.4884, 8.35, 6.15) (-3.2056, 8.35, 4.15) (-2.7056, 8.35, 4.15) (-2.9556, 10, 4.15) (-2.9556, 6.7, 4.15) (0.4884, 8.35, 10.35) (-0.8586, 6.7, 10.35) (-2.2056, 6.7, 8.25) (1.25, 6.7, 8.25) (0.3328, 6.7, 4.15) (-1.2056, 6.7, 1.225) (1.8712, 8.35, 4.15) (-0.7056, 6.7, -1.7) (-1.4556, 6.7, -3.85) (3.45, 0, 7.1276) (3.3693, 0, 8.7924) (2.3295, 0, 11.2513) (3.25, 0, 6.21) (3.05, 0, 5.71) (3.25, 0, 5.21) (50.5444, 6.7, 4.15) (50.5444, 10, 4.15) (50.2944, 8.35, 4.15) (47.1, 8.35, 10.35) (47.1, 8.35, 4.15) on bodies 1
fillet "Fillet11" radius 0.2 1 faces at (43.2397, 0, 10.5333) on bodies 1
equation "d15 = 23.3 mm + 23.8 mm"
named bodies: "Case", "large_pin", "large_pin (1)", "large_pin (2)", "large_pin (3)", "large_pin (4)", "large_pin (5)", "large_pin (6)", "large_pin (7)", "large_pin (8)", "large_pin (9)", "short_pin", "short_pin (1)", "short_pin (2)", "short_pin (3)", "short_pin (4)", "short_pin (5)", "short_pin (6)", "short_pin (7)", "short_pin (8)", "short_pin (9)", "short_pin (10)"
